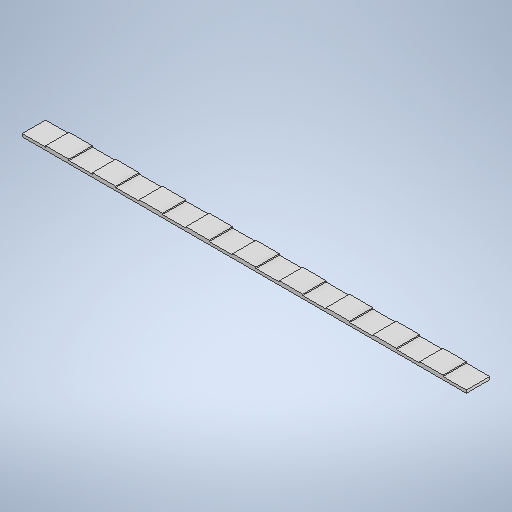
# Autodesk Inventor part: electrodos
Saved by Autodesk Inventor 2025.2 (Build 292293000, 293)
## iProperties
Created: 2025-03-13
Part Number: electrodos
Material: Genérico
Document SubType Name: Modeling
Designer: julia
Density: 1 g/cm^3
Appearance: Valor por defecto
Author: julia
Autodesk Inventor part; units mm, degrees
ref_plane "YZ Plane" through (0, 0, 0) normal (1, 0, 0) x (0, 1, 0)
ref_plane "XZ Plane" through (0, 0, 0) normal (0, 1, 0) x (-1, 0, 0)
ref_plane "XY Plane" through (0, 0, 0) normal (0, 0, 1) x (1, 0, 0)
sketch "Boceto1" plane through (0, 0, 0) normal (0, 0, 1) x (1, 0, 0)
  line L0 (0, 0) -> (17, 0)
  line L1 (17, 0) -> (16.988, 0)
  line L2 (17, 0) -> (17, 0.012)
  line L3 (17, 0.012) -> (16.9, 0.012)
  line L4 (16.9, 0.012) -> (16.9, 0.017)
  line L5 (16.9, 0.017) -> (16.8, 0.017)
  line L6 (16.8, 0.017) -> (16.8, 0.012)
  line L7 (16.8, 0.012) -> (16.7, 0.012)
  line L8 (16.7, 0.012) -> (16.7, 0.017)
  line L9 (16.7, 0.017) -> (16.6, 0.017)
  line L10 (16.6, 0.017) -> (16.6, 0.012)
  line L11 (16.6, 0.012) -> (16.5, 0.012)
  line L12 (16.5, 0.012) -> (16.5, 0.017)
  line L13 (16.5, 0.017) -> (16.4, 0.017)
  line L14 (16.4, 0.017) -> (16.4, 0.012)
  line L15 (16.4, 0.012) -> (16.3, 0.012)
  line L16 (16.3, 0.012) -> (16.3, 0.017)
  line L17 (16.3, 0.017) -> (16.2, 0.017)
  line L18 (16.2, 0.017) -> (16.2, 0.012)
  line L19 (16.2, 0.012) -> (16.1, 0.012)
  line L20 (16.1, 0.012) -> (16.1, 0.017)
  line L21 (16.1, 0.017) -> (16, 0.017)
  line L22 (16, 0.017) -> (16, 0.012)
  line L23 (16, 0.012) -> (15.9, 0.012)
  line L24 (15.9, 0.012) -> (15.9, 0.017)
  line L25 (15.9, 0.017) -> (15.8, 0.017)
  line L26 (15.8, 0.017) -> (15.8, 0.012)
  line L27 (15.8, 0.012) -> (15.7, 0.012)
  line L28 (15.7, 0.012) -> (15.7, 0.017)
  line L29 (15.7, 0.017) -> (15.6, 0.017)
  line L30 (15.6, 0.017) -> (15.6, 0.012)
  line L31 (15.6, 0.012) -> (15.5, 0.012)
  line L32 (15.5, 0.012) -> (15.5, 0.017)
  line L33 (15.5, 0.017) -> (15.4, 0.017)
  line L34 (15.4, 0.017) -> (15.4, 0.012)
  line L35 (15.4, 0.012) -> (15.3, 0.012)
  line L36 (15.3, 0.012) -> (15.3, 0.017)
  line L37 (15.3, 0.017) -> (15.2, 0.017)
  line L38 (15.2, 0.017) -> (15.2, 0.012)
  line L39 (15.2, 0.012) -> (15.1, 0.012)
  line L40 (15.1, 0.012) -> (15.1, 0)
  dimension "d0" = 17
  dimension "d1" = 0.012
  dimension "d2" = 0.012
  dimension "d3" = 0.1
  dimension "d4" = 0.005
  dimension "d5" = 0.1
  dimension "d189" = 0.1
  dimension "d190" = 0.005
  dimension "d191" = 0.1
  dimension "d192" = 0.1
  dimension "d193" = 0.005
  dimension "d194" = 0.1
  dimension "d195" = 0.1
  dimension "d196" = 0.005
  dimension "d197" = 0.1
  dimension "d198" = 0.1
  dimension "d199" = 0.005
  dimension "d200" = 0.1
  dimension "d201" = 0.1
  dimension "d202" = 0.005
  dimension "d203" = 0.1
  dimension "d204" = 0.1
  dimension "d205" = 0.005
  dimension "d206" = 0.1
  dimension "d207" = 0.1
  dimension "d208" = 0.005
  dimension "d209" = 0.1
  dimension "d210" = 0.1
  dimension "d211" = 0.005
  dimension "d212" = 0.1
  dimension "d213" = 0.1
  constraints: 82 end point, 10 horizontal, 2 perpendicular, 2 point on line, 1 parallel, 1 vertical
  measures "d0" distance of L0.start L0.end
  measures "d1" distance of L0.end L1.end
  measures "d2" distance of L0.end L2.end
  measures "d3" distance of L2.end L3.end
  measures "d4" distance of L3.end L4.end
  measures "d5" distance of L4.end L5.end
  measures "d189" distance of L7.start L7.end
  measures "d190" distance of L7.end L8.end
  measures "d191" distance of L8.end L9.end
  measures "d192" distance of L11.start L11.end
  measures "d193" distance of L11.end L12.end
  measures "d194" distance of L12.end L13.end
  measures "d195" distance of L15.start L15.end
  measures "d196" distance of L15.end L16.end
  measures "d197" distance of L16.end L17.end
  measures "d198" distance of L19.start L19.end
  measures "d199" distance of L19.end L20.end
  measures "d200" distance of L20.end L21.end
  measures "d201" distance of L23.start L23.end
  measures "d202" distance of L23.end L24.end
  measures "d203" distance of L24.end L25.end
  measures "d204" distance of L27.start L27.end
  measures "d205" distance of L27.end L28.end
  measures "d206" distance of L28.end L29.end
  measures "d207" distance of L31.start L31.end
  measures "d208" distance of L31.end L32.end
  measures "d209" distance of L32.end L33.end
  measures "d210" distance of L35.start L35.end
  measures "d211" distance of L35.end L36.end
  measures "d212" distance of L36.end L37.end
  measures "d213" distance of L38.end L39.end
extrude "Extrusión1" add sketch "Boceto1" along normal blind 0.1
